Autodesk Fusion 360 part; units mm, degrees
note: some values were not read from the file. Set by a fixed rule: which face or edge a step refers to.
(part 4 of 4)
sketch "Sketch109" plane through (0, 317.5, 0) normal (0, -1, 0) x (1, 0, 0)
  line L0 (-279, 20) -> (-254, 20)
  line L1 (-254, 20) -> (-254, 51.2)
  line L2 (-254, 51.2) -> (-70, 51.2)
  line L3 (-70, 51.2) -> (-70, 76.2)
  line L4 (-70, 76.2) -> (-74.5, 76.2)
  line L5 (-74.5, 76.2) -> (-74.5, 63.7)
  line L6 (-74.5, 63.7) -> (-83.5, 63.7)
  line L7 (-83.5, 63.7) -> (-83.5, 76.2)
  line L8 (-83.5, 76.2) -> (-231.5, 76.2)
  line L9 (-231.5, 76.2) -> (-231.5, 63.7)
  line L10 (-231.5, 63.7) -> (-240.5, 63.7)
  line L11 (-240.5, 63.7) -> (-240.5, 86.2)
  line L12 (-240.5, 86.2) -> (-245, 86.2)
  line L13 (-245, 86.2) -> (-245, 79.7)
  line L14 (-245, 79.7) -> (-314, 79.7)
  line L15 (-314, 79.7) -> (-314, 3)
  line L16 (-314, 3) -> (-279, 3)
  line L17 (-279, 3) -> (-279, 20)
  line L18 (-279, 20) -> (-314, 20)
  line L19 (-314, 20) -> (-314, 3)
  line L20 (-314, 3) -> (-279, 3)
  line L21 (-279, 3) -> (-279, 20)
  constraint horizontal L18
  constraint vertical L19
  constraint horizontal L20
  constraint vertical L21
  constraint coincident L15.end L16.start
  constraint coincident L0.start L17.end
extrude "Extrude276" add sketch "Sketch109" along normal blind 117 separate body contours L15 L16 L17 L18 L19 L20 L21 makes body 17
sketch "Sketch110" plane through (-314, 0, 0) normal (-1, 0, 0) x (0, 0, 1)
  line L0 (20, 317.5) -> (3, 317.5)
  line L1 (3, 317.5) -> (3, 200.5)
  line L2 (3, 200.5) -> (20, 200.5)
  line L3 (20, 200.5) -> (20, 317.5)
  line L4 (20, 200.5) -> (36.1286, 200.5)
  line L5 (36.1286, 200.5) -> (36.1286, 210.5)
  line L6 (36.1286, 210.5) -> (20, 210.5)
  line L7 (20, 210.5) -> (20, 200.5)
  point P0 (36.1286, 210.5)
  constraint horizontal L4
  constraint vertical L5
  constraint horizontal L6
  constraint vertical L7
  constraint coincident P0 L5.end
  constraint coincident L2.end L3.start
extrude "Extrude277" add sketch "Sketch110" against normal blind 35 contours L3 L4 L5 L6 L7 bodies 16 15 17
extrude "Extrude278" cut 1 faces at (-291, 246.1667, 79.7) along direction (0, 0, 1) blind 1 on bodies 16 bodies 16
extrude "Extrude279" cut 1 faces at (-182.1667, 193, 72.0333) along direction (0, 1, 0) blind 7.5 on bodies 16 bodies 16
extrude "Extrude280" add 1 faces at (-294, 210.5, 50.6333) along direction (0, 1, 0) blind 1.5 on bodies 16 bodies 16
extrude "Extrude281" add 1 faces at (-294, 212, 50.6333) along direction (0, 1, 0) blind 2 on bodies 16 bodies 16
extrude "Extrude282" add 1 faces at (-251.6667, 210.5, 15.1667) along direction (0, 1, 0) blind 6.5 on bodies 16 bodies 16
sketch "Sketch111" plane through (-314, 0, 0) normal (-1, 0, 0) x (0, 0, 1)
  line L0 (3, 200.5) -> (86.2, 200.5)
  line L1 (86.2, 200.5) -> (86.2, 333)
  line L2 (86.2, 333) -> (3, 333)
  line L3 (3, 333) -> (3, 200.5)
  line L4 (20, 214) -> (20, 317.5)
  line L5 (20, 317.5) -> (80.7, 317.5)
  line L6 (80.7, 317.5) -> (80.7, 214)
  line L7 (80.7, 214) -> (20, 214)
  line L8 (3, 333) -> (86.2, 333)
  line L9 (86.2, 333) -> (86.2, 200.5)
  line L10 (86.2, 200.5) -> (3, 200.5)
  line L11 (3, 200.5) -> (3, 333)
  constraint horizontal L8
  constraint vertical L9
  constraint horizontal L10
  constraint vertical L11
  constraint coincident L0.end L1.start
  constraint coincident L2.end L3.start
extrude "Extrude283" add sketch "Sketch111" along normal blind 5 separate body contours L0 L1 L2 L3 L8 L9 L10 L11 | L4 L5 L6 L7 makes body 18
extrude "Extrude284" add 1 faces at (-319, 244.6667, 30.7333) along direction (-1, 0, 0) blind 5 on bodies 18 bodies 18
extrude "Extrude285" cut 1 faces at (-294, 249.5, 20) along direction (0, 0, -1) blind 10 on bodies 16 bodies 16
sketch "Sketch112" plane through (0, 0, 0) normal (0, -1, 0) x (1, 0, 0)
  line L0 (-66, -20) -> (-66, -46)
  line L1 (-66, -46) -> (-249, -46)
  line L2 (-249, -46) -> (-249, -20)
  line L3 (-249, -20) -> (-66, -20)
  circle A0 centre (-152, -53.875) radius 4
  circle A1 centre (-163, -12.125) radius 4
  line L4 (-185, 3) -> (-264, 3)
  line L5 (-264, 3) -> (-264, -71)
  line L6 (-264, -71) -> (-56, -71)
  line L7 (-56, -71) -> (-56, 0)
  line L8 (-56, 0) -> (-36, 0)
  line L9 (-36, 0) -> (-36, 36.1286)
  line L10 (-36, 36.1286) -> (-45, 45.1607)
  line L11 (-45, 45.1607) -> (-45, 3)
  line L12 (-45, 3) -> (-130, 3)
  line L13 (-130, 3) -> (-185, 3)
  line L14 (-66, -46) -> (-111, -46)
  line L15 (-111, -46) -> (-111, -20)
  line L16 (-111, -20) -> (-66, -20)
  line L17 (-66, -20) -> (-66, -46)
  line L18 (-249, -46) -> (-204, -46)
  line L19 (-204, -46) -> (-204, -20)
  line L20 (-204, -20) -> (-249, -20)
  line L21 (-249, -20) -> (-249, -46)
  dimension "d708" = 45
  dimension "d709" = 45
  constraint horizontal L14
  constraint vertical L15
  constraint horizontal L16
  constraint vertical L17
  constraint coincident L0.end L1.start
  constraint horizontal L18
  constraint vertical L19
  constraint horizontal L20
  constraint vertical L21
  constraint coincident L1.end L2.start
  measures "d708" distance of L0.end L14.end
  measures "d709" distance of L1.end L18.end
extrude "Extrude286" add sketch "Sketch112" against normal blind 5 separate body contours L0 L1 L3 L14 L15 L16 L17 makes body 19
sketch "Sketch113" plane through (0, 0, 0) normal (0, -1, 0) x (1, 0, 0)
  line L0 (-66, -20) -> (-66, -46)
  line L1 (-66, -46) -> (-249, -46)
  line L2 (-249, -46) -> (-249, -20)
  line L3 (-249, -20) -> (-66, -20)
  circle A0 centre (-152, -53.875) radius 4
  circle A1 centre (-163, -12.125) radius 4
  line L4 (-185, 3) -> (-264, 3)
  line L5 (-264, 3) -> (-264, -71)
  line L6 (-264, -71) -> (-56, -71)
  line L7 (-56, -71) -> (-56, 0)
  line L8 (-56, 0) -> (-36, 0)
  line L9 (-36, 0) -> (-36, 36.1286)
  line L10 (-36, 36.1286) -> (-45, 45.1607)
  line L11 (-45, 45.1607) -> (-45, 3)
  line L12 (-45, 3) -> (-130, 3)
  line L13 (-130, 3) -> (-185, 3)
  line L14 (-249, -20) -> (-204, -20)
  line L15 (-204, -20) -> (-204, -46)
  line L16 (-204, -46) -> (-249, -46)
  line L17 (-249, -46) -> (-249, -20)
  dimension "d712" = 45
  constraint horizontal L14
  constraint vertical L15
  constraint horizontal L16
  constraint vertical L17
  constraint coincident L2.end L3.start
  measures "d712" distance of L2.end L14.end
extrude "Extrude287" add sketch "Sketch113" against normal blind 5 separate body contours L1 L2 L3 L14 L15 L16 L17 makes body 20
sketch "Sketch114" plane through (0, 0, 0) normal (0, 0, -1) x (-1, 0, 0)
  line L0 (36, 333) -> (36, 0)
  line L1 (36, 0) -> (56, 0)
  line L2 (56, 0) -> (56, 328)
  line L3 (56, 328) -> (56, 333)
  line L4 (56, 333) -> (36, 333)
  line L5 (36, 333) -> (56, 333)
  line L6 (56, 333) -> (56, 328)
  line L7 (56, 328) -> (36, 328)
  line L8 (36, 328) -> (36, 333)
  line L9 (56, 328) -> (49.25, 328)
  line L10 (49.25, 328) -> (49.25, 304.4)
  line L11 (49.25, 304.4) -> (56, 304.4)
  line L12 (56, 304.4) -> (56, 328)
  line L13 (49.25, 328) -> (42.75, 328)
  line L14 (42.75, 328) -> (42.75, 304.4)
  line L15 (42.75, 304.4) -> (49.25, 304.4)
  line L16 (49.25, 304.4) -> (49.25, 328)
  dimension "d715" = 6.75
  dimension "d716" = 23.6
  dimension "d717" = 6.5
  constraint horizontal L5
  constraint vertical L6
  constraint horizontal L7
  constraint vertical L8
  constraint coincident L2.end L3.start
  constraint coincident L0.start L4.end
  constraint horizontal L9
  constraint vertical L10
  constraint horizontal L11
  constraint vertical L12
  constraint horizontal L13
  constraint vertical L14
  constraint horizontal L15
  constraint vertical L16
  measures "d715" distance of L2.end L9.end
  measures "d716" distance of L2.end L11.end
  measures "d717" distance of L9.end L13.end
extrude "Extrude288" cut sketch "Sketch114" against normal blind 28 contours L7 L10 L13 L14 L15 L16 bodies 16
sketch "Sketch115" plane through (-56, 0, 0) normal (-1, 0, 0) x (0, 0, 1)
  line L0 (0, 333) -> (0, 328)
  line L1 (0, 328) -> (61.2, 328)
  line L2 (61.2, 328) -> (61.2, 333)
  line L3 (61.2, 333) -> (0, 333)
extrude "Extrude289" cut 1 faces at (-44.9167, 320.1333, 28) along direction (0, 0, 1) blind 5 on bodies 16 bodies 16
sketch "Sketch116" plane through (-61, 0, 0) normal (-1, 0, 0) x (0, 0, 1)
  line L0 (28, 328) -> (33, 328)
  line L1 (33, 328) -> (33, 323)
  line L2 (33, 323) -> (28, 323)
  line L3 (28, 323) -> (28, 328)
  line L4 (28, 323) -> (33, 323)
  line L5 (33, 323) -> (33, 304.4)
  line L6 (33, 304.4) -> (28, 304.4)
  line L7 (28, 304.4) -> (28, 323)
  point P0 (28, 328)
  point P1 (33, 304.4)
  dimension "d725" = 5
  constraint horizontal L0
  constraint vertical L1
  constraint horizontal L2
  constraint vertical L3
  constraint coincident P0 L0.start
  constraint horizontal L4
  constraint vertical L5
  constraint horizontal L6
  constraint vertical L7
  constraint coincident P1 L5.end
  measures "d725" distance of P0 L2.end
extrude "Extrude290" cut sketch "Sketch116" against normal blind 18.25 contours L2 L4 L5 L6 L7 bodies 16
extrude "Extrude291" cut 1 faces at (-245, 70, -59.6667) along direction (0, -1, 0) blind 8 on bodies 16 bodies 16
sketch "Sketch117" plane through (-61, 0, 0) normal (-1, 0, 0) x (0, 0, 1)
  line L0 (0, 304.4) -> (13, 304.4)
  line L1 (13, 304.4) -> (13, 313.4)
  line L2 (13, 313.4) -> (0, 313.4)
  line L3 (0, 313.4) -> (0, 304.4)
  circle A0 centre (13, 313.4) radius 1.375
  point P0 (0, 304.4)
  dimension "d730" = 13
  dimension "d731" = 9
  dimension "d732" = 2.75
  constraint horizontal L0
  constraint vertical L1
  constraint horizontal L2
  constraint vertical L3
  constraint coincident P0 L0.start
  constraint coincident L1.end L2.start
  measures "d730" distance of P0 L0.end
  measures "d731" distance of P0 L2.end
  measures "d732" diameter of A0
extrude "Extrude292" cut sketch "Sketch117" against normal blind 11.75 contours L1 L2 A0 | L1 L2 A0 bodies 16
sketch "Sketch118" plane through (-61, 0, 0) normal (-1, 0, 0) x (0, 0, 1)
  circle A0 centre (13, 313.4) radius 1.375
  circle A1 centre (13, 313.4) radius 1.375
  line L0 (13, 313.4) -> (0, 313.4)
  line L1 (0, 313.4) -> (0, 322.9)
  line L2 (0, 322.9) -> (13, 322.9)
  line L3 (13, 322.9) -> (13, 313.4)
  line L4 (0, 304.4) -> (0, 328)
  circle A2 centre (13, 322.9) radius 1.375
  dimension "d735" = 9.5
  dimension "d736" = 2.75
  constraint concentric A0 A1
  constraint horizontal L0
  constraint vertical L1
  constraint horizontal L2
  constraint vertical L3
  constraint coincident L1.end L4
  constraint coincident A0.centre A1.centre
  constraint coincident L2.end L3.start
  measures "d735" distance of A0.centre L2.end
  measures "d736" diameter of A2
extrude "Extrude293" cut sketch "Sketch118" against normal blind 11.75 contours L2 L3 A2 | L2 L3 A2 bodies 16
sketch "Sketch119" plane through (-61, 0, 0) normal (-1, 0, 0) x (0, 0, 1)
  circle A0 centre (13, 322.9) radius 1.375
  circle A1 centre (13, 322.9) radius 1.375
  circle A2 centre (13, 313.4) radius 1.375
  circle A3 centre (13, 313.4) radius 1.375
  circle A4 centre (13, 322.9) radius 2.375
  circle A5 centre (13, 313.4) radius 2.375
  dimension "d739" = 1
  dimension "d740" = 1
  constraint concentric A0 A1
  constraint concentric A2 A3
extrude "Extrude294" cut sketch "Sketch119" against normal blind 4 bodies 16
extrude "Extrude295" add 1 faces at (-294, 248.5, 10) along direction (0, 0, 1) blind 20 on bodies 16 bodies 16 18
sketch "Sketch120" plane through (0, 200.5, 0) normal (0, -1, 0) x (1, 0, 0)
  line L0 (-279, 3) -> (-279, 36.1286)
  line L1 (-279, 36.1286) -> (-270, 45.1607)
  line L2 (-270, 45.1607) -> (-270, 56.2)
  line L3 (-270, 56.2) -> (-254, 76.2)
  line L4 (-254, 76.2) -> (-254, 56.2)
  line L5 (-254, 56.2) -> (-61, 56.2)
  line L6 (-61, 56.2) -> (-61, 76.2)
  line L7 (-61, 76.2) -> (-74.5, 76.2)
  line L8 (-74.5, 76.2) -> (-74.5, 63.7)
  line L9 (-74.5, 63.7) -> (-83.5, 63.7)
  line L10 (-83.5, 63.7) -> (-83.5, 76.2)
  line L11 (-83.5, 76.2) -> (-231.5, 76.2)
  line L12 (-231.5, 76.2) -> (-231.5, 63.7)
  line L13 (-231.5, 63.7) -> (-240.5, 63.7)
  line L14 (-240.5, 63.7) -> (-240.5, 86.2)
  line L15 (-240.5, 86.2) -> (-324, 86.2)
  line L16 (-324, 86.2) -> (-324, 3)
  line L17 (-324, 3) -> (-279, 3)
  line L18 (-279, 36.1286) -> (-324, 36.1286)
  line L19 (-324, 36.1286) -> (-324, 3)
  line L20 (-324, 3) -> (-279, 3)
  line L21 (-279, 3) -> (-279, 36.1286)
  constraint horizontal L18
  constraint vertical L19
  constraint horizontal L20
  constraint vertical L21
  constraint coincident L16.end L17.start
  constraint coincident L0.end L1.start
extrude "Extrude296" cut sketch "Sketch120" against normal blind 140 contours L0 L16 L17 L18 L19 L20 L21 bodies 16
extrude "Extrude297" add 1 faces at (-305.6667, 327.8333, 36.1286) along direction (0, 0, -1) blind 6.129 on bodies 16 bodies 16
sketch "Sketch121" plane through (0, 0, 29.9996) normal (0, 0, -1) x (-1, 0, 0)
  line L0 (324, 333) -> (279, 333)
  line L1 (279, 333) -> (279, 317.5)
  line L2 (279, 317.5) -> (314, 317.5)
  line L3 (314, 317.5) -> (314, 214)
  line L4 (314, 214) -> (279, 214)
  line L5 (279, 214) -> (279, 200.5)
  line L6 (279, 200.5) -> (324, 200.5)
  line L7 (324, 200.5) -> (324, 333)
  line L8 (279, 333) -> (324, 333)
  line L9 (324, 333) -> (324, 200.5)
  line L10 (324, 200.5) -> (279, 200.5)
  line L11 (279, 200.5) -> (279, 333)
  constraint horizontal L8
  constraint vertical L9
  constraint horizontal L10
  constraint vertical L11
  constraint coincident L6.end L7.start
  constraint coincident L0.end L1.start
extrude "Extrude298" add sketch "Sketch121" along normal blind 5 separate body makes body 21
sketch "Sketch122" plane through (0, 333, 0) normal (0, 1, 0) x (-1, 0, 0)
  line L0 (279, 3) -> (279, 29.9996)
  line L1 (279, 29.9996) -> (324, 29.9996)
  line L2 (324, 29.9996) -> (324, 86.2)
  line L3 (324, 86.2) -> (240.5, 86.2)
  line L4 (240.5, 86.2) -> (240.5, 63.7)
  line L5 (240.5, 63.7) -> (231.5, 63.7)
  line L6 (231.5, 63.7) -> (231.5, 76.2)
  line L7 (231.5, 76.2) -> (83.5, 76.2)
  line L8 (83.5, 76.2) -> (83.5, 63.7)
  line L9 (83.5, 63.7) -> (74.5, 63.7)
  line L10 (74.5, 63.7) -> (74.5, 76.2)
  line L11 (74.5, 76.2) -> (61, 76.2)
  line L12 (61, 76.2) -> (45, 56.1607)
  line L13 (45, 56.1607) -> (53.7273, 56.1821)
  line L14 (53.7273, 56.1821) -> (51, 56.1607)
  line L15 (51, 56.1607) -> (45, 56.1607)
  line L16 (45, 56.1607) -> (45, 45.1607)
  line L17 (45, 45.1607) -> (36, 36.1286)
  line L18 (36, 36.1286) -> (36, 0)
  line L19 (36, 0) -> (56, 0)
  line L20 (56, 0) -> (56, 61.2)
  line L21 (56, 61.2) -> (259, 61.2)
  line L22 (259, 61.2) -> (259, -71)
  line L23 (259, -71) -> (264, -71)
  line L24 (264, -71) -> (264, 3)
  line L25 (264, 3) -> (279, 3)
  line L26 (324, 24.9996) -> (259, 24.9996)
  line L27 (259, 24.9996) -> (259, 86.2)
  line L28 (259, 86.2) -> (324, 86.2)
  line L29 (324, 86.2) -> (324, 24.9996)
  line L30 (324, 86.2) -> (291.5, 86.2)
  line L31 (291.5, 86.2) -> (291.5, 58.1)
  line L32 (291.5, 58.1) -> (324, 58.1)
  line L33 (324, 58.1) -> (324, 86.2)
  line L34 (324, 86.2) -> (307.75, 86.2)
  line L35 (307.75, 86.2) -> (307.75, 72.15)
  line L36 (307.75, 72.15) -> (324, 72.15)
  line L37 (324, 72.15) -> (324, 86.2)
  line L38 (324, 86.2) -> (317, 86.2)
  line L39 (317, 86.2) -> (317, 79.2)
  line L40 (317, 79.2) -> (324, 79.2)
  line L41 (324, 79.2) -> (324, 86.2)
  line L42 (324, 79.2) -> (317, 86.2)
  point P0 (324, 24.9996)
  dimension "d751" = 65
  dimension "d752" = 28.1
  dimension "d753" = 14.05
  dimension "d754" = 7
  dimension "d755" = 7
  constraint horizontal L26
  constraint vertical L27
  constraint horizontal L28
  constraint vertical L29
  constraint coincident L3 L27.end
  constraint coincident P0 L26.start
  constraint horizontal L30
  constraint vertical L31
  constraint horizontal L32
  constraint vertical L33
  constraint coincident L2.end L3.start
  constraint horizontal L34
  constraint vertical L35
  constraint horizontal L36
  constraint vertical L37
  constraint horizontal L38
  constraint vertical L39
  constraint horizontal L40
  constraint vertical L41
  measures "d751" distance of P0 L26.end
  measures "d752" distance of L2.end L32.end
  measures "d753" distance of L2.end L36.end
  measures "d754" distance of L2.end L38.end
  measures "d755" distance of L2.end L40.end
extrude "Extrude299" cut sketch "Sketch122" against normal blind 200 contours L2 L3 L28 L29 L30 L33 L34 L37 L38 L41 L42 bodies 16
sketch "Sketch123" plane through (0, 0, -71) normal (0, 0, -1) x (-1, 0, 0)
  line L0 (259, 333) -> (259, 328)
  line L1 (259, 328) -> (254, 328)
  line L2 (254, 328) -> (254, 25)
  line L3 (254, 25) -> (61, 25)
  line L4 (61, 25) -> (61, 328)
  line L5 (61, 328) -> (56, 328)
  line L6 (56, 328) -> (56, 0)
  line L7 (56, 0) -> (264, 0)
  line L8 (264, 0) -> (264, 333)
  line L9 (264, 333) -> (259, 333)
extrude "Extrude300" add sketch "Sketch123" along normal blind 5 separate body makes body 22
sketch "Sketch124" plane through (-61, 0, 0) normal (-1, 0, 0) x (0, 0, 1)
  circle A0 centre (13, 322.9) radius 2.375
  circle A1 centre (13, 313.4) radius 2.375
  line L0 (33, 323) -> (33, 304.4)
  line L1 (33, 304.4) -> (28, 304.4)
  line L2 (28, 304.4) -> (28, 323)
  line L3 (28, 323) -> (33, 323)
  line L4 (51.2, 5) -> (51.2, 328)
  line L5 (51.2, 328) -> (-71, 328)
  line L6 (-71, 328) -> (-71, 25)
  line L7 (-71, 25) -> (-66, 25)
  line L8 (-66, 25) -> (-66, 217)
  line L9 (-66, 217) -> (-56, 217)
  line L10 (-56, 217) -> (-56, 62)
  line L11 (-56, 62) -> (10, 62)
  line L12 (10, 62) -> (10, 217)
  line L13 (10, 217) -> (20, 217)
  line L14 (20, 217) -> (20, 5)
  line L15 (20, 5) -> (51.2, 5)
extrude "Extrude301" add 1 faces at (-254, 70.1667, 62.8667) along direction (1, 0, 0) blind 10 on bodies 16 bodies 16
extrude "Extrude302" add 1 faces at (-61, 135.3333, 69.5333) along direction (-1, 0, 0) blind 10 on bodies 16 bodies 16
extrude "Extrude303" add 1 faces at (-246.0289, 146, 30.2696) along direction (0, 1, 0) blind 5 on bodies 16 bodies 16
extrude "Extrude304" add 1 faces at (-229.0289, 146, 34.1304) along direction (0, 1, 0) blind 5 on bodies 16 bodies 16
extrude "Extrude305" add 1 faces at (-240.8138, 142, 39.8515) along direction (0, 1, 0) blind 5 on bodies 16 bodies 16
extrude "Extrude306" cut 1 faces at (-235.9784, 135, 39.5909) along direction (0, 1, 0) blind 5 on bodies 16 bodies 16
sketch "Sketch125" plane through (0, 155, 0) normal (0, 1, 0) x (-1, 0, 0)
  line L0 (254, 10) -> (254, 51.2)
  line L1 (254, 51.2) -> (250.5, 51.2)
  line L2 (250.5, 51.2) -> (250.5, 28.7)
  line L3 (250.5, 28.7) -> (226.5, 28.7)
  line L4 (226.5, 28.7) -> (226.5, 51.2)
  line L5 (226.5, 51.2) -> (219, 51.2)
  line L6 (219, 51.2) -> (219, 41.8)
  line L7 (219, 41.8) -> (213.5, 41.8)
  line L8 (213.5, 41.8) -> (213.5, 37.3)
  line L9 (213.5, 37.3) -> (223, 37.3)
  line L10 (223, 37.3) -> (223, 20)
  line L11 (223, 20) -> (236, 20)
  line L12 (236, 20) -> (236, 10)
  line L13 (236, 10) -> (241, 10)
  line L14 (241, 10) -> (241, 15.5)
  line L15 (241, 15.5) -> (247, 15.5)
  line L16 (247, 15.5) -> (247, 10)
  line L17 (247, 10) -> (254, 10)
  line L18 (236, 20) -> (254, 20)
  line L19 (254, 20) -> (254, 10)
  line L20 (254, 10) -> (236, 10)
  line L21 (236, 10) -> (236, 20)
  constraint horizontal L18
  constraint vertical L19
  constraint horizontal L20
  constraint vertical L21
  constraint coincident L0.start L17.end
  constraint coincident L11.end L12.start
extrude "Extrude307" add sketch "Sketch125" along normal blind 62 separate body contours L0 L12 L13 L14 L15 L16 L17 L18 L19 L20 L21 makes body 23
sketch "Sketch126" plane through (0, 333, 0) normal (0, 1, 0) x (-1, 0, 0)
  line L0 (324, 79.2) -> (317, 86.2)
  line L1 (317, 86.2) -> (240.5, 86.2)
  line L2 (240.5, 86.2) -> (240.5, 63.7)
  line L3 (240.5, 63.7) -> (231.5, 63.7)
  line L4 (231.5, 63.7) -> (231.5, 76.2)
  line L5 (231.5, 76.2) -> (83.5, 76.2)
  line L6 (83.5, 76.2) -> (83.5, 63.7)
  line L7 (83.5, 63.7) -> (74.5, 63.7)
  line L8 (74.5, 63.7) -> (74.5, 76.2)
  line L9 (74.5, 76.2) -> (61, 76.2)
  line L10 (61, 76.2) -> (45, 56.1607)
  line L11 (45, 56.1607) -> (53.7273, 56.1821)
  line L12 (53.7273, 56.1821) -> (51, 56.1607)
  line L13 (51, 56.1607) -> (45, 56.1607)
  line L14 (45, 56.1607) -> (45, 45.1607)
  line L15 (45, 45.1607) -> (36, 36.1286)
  line L16 (36, 36.1286) -> (36, 0)
  line L17 (36, 0) -> (56, 0)
  line L18 (56, 0) -> (56, 61.2)
  line L19 (56, 61.2) -> (259, 61.2)
  line L20 (259, 61.2) -> (259, -71)
  line L21 (259, -71) -> (264, -71)
  line L22 (264, -71) -> (264, 3)
  line L23 (264, 3) -> (279, 3)
  line L24 (279, 3) -> (279, 29.9996)
  line L25 (279, 29.9996) -> (324, 29.9996)
  line L26 (324, 29.9996) -> (324, 79.2)
  line L27 (264, 3) -> (259, 3)
  line L28 (259, 3) -> (259, -76)
  line L29 (259, -76) -> (264, -76)
  line L30 (264, -76) -> (264, 3)
  point P0 (259, -76)
  constraint horizontal L27
  constraint vertical L28
  constraint horizontal L29
  constraint vertical L30
  constraint coincident P0 L28.end
  constraint coincident L22.end L23.start
extrude "Extrude308" cut sketch "Sketch126" against normal blind 5 contours L20 L21 L22 L27 L28 L30 bodies 16
extrude "Extrude309" cut 1 faces at (-262.3333, 333, -72.6667) along direction (0, -1, 0) blind 5 on bodies 22 bodies 22
extrude "Extrude310" cut 1 faces at (-264, 179.5, -46.4333) along direction (1, 0, 0) blind 5 on bodies 16 bodies 16
extrude "Extrude311" cut 1 faces at (-264, 109.3333, -72.6667) along direction (1, 0, 0) blind 5 on bodies 22 bodies 22
sketch "Sketch127" plane through (0, 0, 3) normal (0, 0, -1) x (-1, 0, 0)
  line L0 (279, 0) -> (279, 333)
  line L1 (279, 333) -> (259, 333)
  line L2 (259, 333) -> (259, 328)
  line L3 (259, 328) -> (259, 317.5)
  line L4 (259, 317.5) -> (254, 317.5)
  line L5 (254, 317.5) -> (254, 210.5)
  line L6 (254, 210.5) -> (259, 210.5)
  line L7 (259, 210.5) -> (259, 0)
  line L8 (259, 0) -> (185, 0)
  line L9 (185, 0) -> (185, -3)
  line L10 (185, -3) -> (270, -3)
  line L11 (270, -3) -> (270, 0)
  line L12 (270, 0) -> (279, 0)
  line L13 (259, 0) -> (279, 0)
  line L14 (279, 0) -> (279, 333)
  line L15 (279, 333) -> (259, 333)
  line L16 (259, 333) -> (259, 0)
  constraint horizontal L13
  constraint vertical L14
  constraint horizontal L15
  constraint vertical L16
  constraint coincident L0.end L1.start
  constraint coincident L7.end L8.start
extrude "Extrude312" add sketch "Sketch127" along normal blind 3 separate body contours L0 L1 L2 L3 L7 L12 L13 L14 L15 L16 makes body 24
sketch "Sketch128" plane through (0, 333, 0) normal (0, 1, 0) x (-1, 0, 0)
  line L0 (259, 3) -> (279, 3)
  line L1 (279, 3) -> (279, 29.9996)
  line L2 (279, 29.9996) -> (324, 29.9996)
  line L3 (324, 29.9996) -> (324, 79.2)
  line L4 (324, 79.2) -> (317, 86.2)
  line L5 (317, 86.2) -> (240.5, 86.2)
  line L6 (240.5, 86.2) -> (240.5, 63.7)
  line L7 (240.5, 63.7) -> (231.5, 63.7)
  line L8 (231.5, 63.7) -> (231.5, 76.2)
  line L9 (231.5, 76.2) -> (83.5, 76.2)
  line L10 (83.5, 76.2) -> (83.5, 63.7)
  line L11 (83.5, 63.7) -> (74.5, 63.7)
  line L12 (74.5, 63.7) -> (74.5, 76.2)
  line L13 (74.5, 76.2) -> (61, 76.2)
  line L14 (61, 76.2) -> (45, 56.1607)
  line L15 (45, 56.1607) -> (53.7273, 56.1821)
  line L16 (53.7273, 56.1821) -> (51, 56.1607)
  line L17 (51, 56.1607) -> (45, 56.1607)
  line L18 (45, 56.1607) -> (45, 45.1607)
  line L19 (45, 45.1607) -> (36, 36.1286)
  line L20 (36, 36.1286) -> (36, 0)
  line L21 (36, 0) -> (56, 0)
  line L22 (56, 0) -> (56, 61.2)
  line L23 (56, 61.2) -> (259, 61.2)
  line L24 (259, 61.2) -> (259, 3)
  line L25 (56, 61.2) -> (74.5, 61.2)
  line L26 (74.5, 61.2) -> (74.5, 76.2)
  line L27 (74.5, 76.2) -> (56, 76.2)
  line L28 (56, 76.2) -> (56, 61.2)
  line L29 (56, 61.2) -> (56, 76.2)
  line L30 (56, 76.2) -> (51, 76.2)
  line L31 (51, 76.2) -> (51, 61.2)
  line L32 (51, 61.2) -> (56, 61.2)
  line L33 (56, 61.2) -> (56, 76.2)
  line L34 (51, 63.6754) -> (61, 76.2)
  line L35 (51, 61.2) -> (74.5, 61.2)
  line L36 (240.5, 76.2) -> (264, 76.2)
  line L37 (264, 76.2) -> (264, 61.2)
  line L38 (264, 61.2) -> (240.5, 61.2)
  line L39 (240.5, 61.2) -> (240.5, 76.2)
  dimension "d784" = 5
  dimension "d785" = 23.5
  constraint horizontal L25
  constraint vertical L26
  constraint horizontal L27
  constraint vertical L28
  constraint coincident L12.end L13.start
  constraint coincident L22.end L23.start
  constraint vertical L29
  constraint horizontal L30
  constraint vertical L31
  constraint horizontal L32
  constraint vertical L33
  constraint coincident L14 L34.start
  constraint coincident L31 L34.start
  constraint coincident L13.end L14.start
  constraint perpendicular L26 L35
  constraint horizontal L36
  constraint vertical L37
  constraint horizontal L38
  constraint vertical L39
  constraint coincident L6 L36.start
  measures "d784" distance of L27.end L30.end
  measures "d785" distance of L36.start L36.end
extrude "Extrude313" add sketch "Sketch128" along normal blind 5 separate body contours L0 L1 L2 L3 L4 L5 L6 L24 L36 L37 L38 makes body 25
sketch "Sketch129" plane through (0, 333, 0) normal (0, 1, 0) x (-1, 0, 0)
  line L0 (259, 3) -> (279, 3)
  line L1 (279, 3) -> (279, 29.9996)
  line L2 (279, 29.9996) -> (324, 29.9996)
  line L3 (324, 29.9996) -> (324, 79.2)
  line L4 (324, 79.2) -> (317, 86.2)
  line L5 (317, 86.2) -> (240.5, 86.2)
  line L6 (240.5, 86.2) -> (240.5, 63.7)
  line L7 (240.5, 63.7) -> (231.5, 63.7)
  line L8 (231.5, 63.7) -> (231.5, 76.2)
  line L9 (231.5, 76.2) -> (83.5, 76.2)
  line L10 (83.5, 76.2) -> (83.5, 63.7)
  line L11 (83.5, 63.7) -> (74.5, 63.7)
  line L12 (74.5, 63.7) -> (74.5, 76.2)
  line L13 (74.5, 76.2) -> (61, 76.2)
  line L14 (61, 76.2) -> (45, 56.1607)
  line L15 (45, 56.1607) -> (53.7273, 56.1821)
  line L16 (53.7273, 56.1821) -> (51, 56.1607)
  line L17 (51, 56.1607) -> (45, 56.1607)
  line L18 (45, 56.1607) -> (45, 45.1607)
  line L19 (45, 45.1607) -> (36, 36.1286)
  line L20 (36, 36.1286) -> (36, 0)
  line L21 (36, 0) -> (56, 0)
  line L22 (56, 0) -> (56, 61.2)
  line L23 (56, 61.2) -> (259, 61.2)
  line L24 (259, 61.2) -> (259, 3)
  line L25 (49.0235, 61.2) -> (74.5, 61.2)
  line L26 (74.5, 61.2) -> (74.5, 76.2)
  line L27 (74.5, 76.2) -> (49.0235, 76.2)
  line L28 (49.0235, 76.2) -> (49.0235, 61.2)
  line L29 (56, 61.2) -> (51, 61.2)
  line L30 (51, 61.2) -> (51, 76.2)
  line L31 (51, 76.2) -> (56, 76.2)
  line L32 (56, 76.2) -> (56, 61.2)
  line L33 (51, 63.6754) -> (61, 76.2)
  dimension "d788" = 5
  constraint horizontal L25
  constraint vertical L26
  constraint horizontal L27
  constraint vertical L28
  constraint coincident L12.end L13.start
  constraint coincident L14 L25.start
  constraint horizontal L29
  constraint vertical L30
  constraint horizontal L31
  constraint vertical L32
  constraint coincident L22.end L23.start
  constraint coincident L14 L33.start
  constraint coincident L30 L33.start
  constraint coincident L13.end L14.start
  measures "d788" distance of L22.end L29.end
extrude "Extrude314" add sketch "Sketch129" along normal blind 5 separate body contours L14 L18 L19 L20 L21 L22 L25 L29 makes body 26
extrude "Extrude315" add 1 faces at (-265.6667, 334.6667, 3) along direction (0, 0, -1) blind 3 on bodies 25 bodies 25 19 20 21 22 23 26 16 24
extrude "Extrude316" add 1 faces at (-309, 333, 28.3329) along direction (0, 1, 0) blind 5 on bodies 21 bodies 21 26 25
extrude "Extrude317" cut 1 faces at (-56, 334.6667, 20.4) along direction (1, 0, 0) blind 5 on bodies 26 bodies 26
sketch "Sketch130" plane through (0, 333, 0) normal (0, 1, 0) x (-1, 0, 0)
  line L0 (259, 61.2) -> (264, 61.2)
  line L1 (264, 61.2) -> (264, 76.2)
  line L2 (264, 76.2) -> (240.5, 76.2)
  line L3 (240.5, 76.2) -> (240.5, 63.7)
  line L4 (240.5, 63.7) -> (231.5, 63.7)
  line L5 (231.5, 63.7) -> (231.5, 76.2)
  line L6 (231.5, 76.2) -> (83.5, 76.2)
  line L7 (83.5, 76.2) -> (83.5, 63.7)
  line L8 (83.5, 63.7) -> (74.5, 63.7)
  line L9 (74.5, 63.7) -> (74.5, 76.2)
  line L10 (74.5, 76.2) -> (61, 76.2)
  line L11 (61, 76.2) -> (45, 56.1607)
  line L12 (51, 56.1607) -> (45, 56.1607)
  line L13 (45, 56.1607) -> (45, 45.1607)
  line L14 (45, 45.1607) -> (36, 36.1286)
  line L15 (36, 36.1286) -> (36, 0)
  line L16 (36, 0) -> (56, 0)
  line L17 (56, 0) -> (56, 61.2)
  line L18 (56, 61.2) -> (259, 61.2)
  line L19 (56, 0, -5) -> (36, 0, -5)
  line L20 (36, 0, -5) -> (36, 0, 5)
  line L21 (36, 0, 5) -> (56, 0, 5)
  line L22 (56, 0, 5) -> (56, 0, -5)
  line L23 (36, 0, 5) -> (51, 0, 5)
  line L24 (36, 0, -5) -> (43.5, 0, 5)
  line L25 (259, 0, -5) -> (279, 0, -5)
  line L26 (279, 0, -5) -> (279, 0, 5)
  line L27 (279, 0, 5) -> (259, 0, 5)
  line L28 (259, 0, 5) -> (259, 0, -5)
  line L29 (279, 0, -5) -> (269, 0, 5)
  point P0 (56, 0)
  point P1 (36, 0)
  point P2 (259, 0)
  point P3 (279, 0)
  constraint coincident P1 L15.end
  constraint coincident P0 L16.end
extrude "Extrude318" cut sketch "Sketch130" along normal blind 25 contours L16 L20 L24 | L16 L20 L21 L23 L24 | L26 L27 L29 in plane through (0, 333, 0) normal (0, 0, 1) bodies 21 26
extrude "Extrude319" cut 1 faces at (-39.75, 336.3333, 25) along direction (0, 0, 1) blind 21 on bodies 26 bodies 26
extrude "Extrude320" cut 1 faces at (-37.25, 331.3333, 25) along direction (0, 0, 1) blind 19 on bodies 21 bodies 21
sketch "Sketch131" plane through (-259, 0, 0) normal (1, 0, 0) x (0, 0, -1)
  line L0 (0, 338) -> (-61.2, 338)
  line L1 (-61.2, 338) -> (-61.2, 333)
  line L2 (-61.2, 333) -> (-61.2, 328)
  line L3 (-61.2, 328) -> (0, 328)
  line L4 (0, 328) -> (0, 338)
  line L5 (0, 338) -> (-61.2, 338)
  line L6 (-61.2, 338) -> (-61.2, 333)
  line L7 (-61.2, 333) -> (0, 333)
  line L8 (0, 333) -> (0, 338)
  constraint horizontal L5
  constraint vertical L6
  constraint horizontal L7
  constraint vertical L8
  constraint coincident L1.end L2.start
  constraint coincident L0.start L4.end
extrude "Extrude321" cut sketch "Sketch131" against normal blind 5 contours L0 L1 L4 L5 L6 L7 L8 bodies 21
sketch "Sketch132" plane through (0, 338, 0) normal (0, 1, 0) x (-1, 0, 0)
  line L0 (264, 76.2) -> (264, 0)
  line L1 (264, 0) -> (269, 0)
  line L2 (269, 0) -> (269, 25)
  line L3 (269, 25) -> (279, 25)
  line L4 (279, 25) -> (279, 24.9996)
  line L5 (279, 24.9996) -> (324, 24.9996)
  line L6 (324, 24.9996) -> (324, 79.2)
  line L7 (324, 79.2) -> (317, 86.2)
  line L8 (317, 86.2) -> (240.5, 86.2)
  line L9 (240.5, 86.2) -> (240.5, 76.2)
  line L10 (240.5, 76.2) -> (264, 76.2)
  line L11 (324, 24.9996) -> (317, 24.9996)
  line L12 (317, 24.9996) -> (317, 31.9996)
  line L13 (317, 31.9996) -> (324, 31.9996)
  line L14 (324, 31.9996) -> (324, 24.9996)
  line L15 (317, 24.9996) -> (324, 31.9996)
  dimension "d807" = 7
  dimension "d808" = 7
  constraint horizontal L11
  constraint vertical L12
  constraint horizontal L13
  constraint vertical L14
  constraint coincident L5.end L6.start
  measures "d807" distance of L5.end L11.end
  measures "d808" distance of L5.end L13.end
extrude "Extrude322" cut sketch "Sketch132" against normal blind 140 contours L5 L6 L11 L14 L15 bodies 21
sketch "Sketch133" plane through (0, 0, 0) normal (0, 0, -1) x (-1, 0, 0)
  line L0 (43.5, 338) -> (39.75, 333)
  line L1 (39.75, 333) -> (51, 333)
  line L2 (51, 333) -> (51, 338)
  line L3 (51, 338) -> (43.5, 338)
  line L4 (39.75, 333) -> (42.65, 333)
  line L5 (42.65, 333) -> (42.65, 338)
  line L6 (42.65, 338) -> (39.75, 338)
  line L7 (39.75, 338) -> (39.75, 333)
  line L8 (42.65, 333) -> (51, 333)
  line L9 (51, 333) -> (51, 338)
  line L10 (51, 338) -> (42.65, 338)
  line L11 (42.65, 338) -> (42.65, 333)
  line L12 (51, 333) -> (46, 333)
  line L13 (46, 333) -> (46, 338)
  line L14 (46, 338) -> (51, 338)
  line L15 (51, 338) -> (51, 333)
  line L16 (46, 338) -> (51, 338)
  line L17 (51, 338, 0) -> (51, 338, -61.2)
  line L18 (51, 338, -61.2) -> (46, 338, -61.2)
  line L19 (46, 338, -61.2) -> (46, 338, 0)
  line L20 (46, 338) -> (51, 338)
  line L21 (51, 338) -> (51, 343)
  line L22 (51, 343) -> (46, 343)
  line L23 (46, 343) -> (46, 338)
  line L24 (51, 343) -> (46, 338)
  point P0 (51, 338)
  dimension "d811" = 2.9
  dimension "d812" = 5
  dimension "d813" = 5
  constraint horizontal L4
  constraint vertical L5
  constraint horizontal L6
  constraint vertical L7
  constraint coincident L0.end L1.start
  constraint horizontal L8
  constraint vertical L9
  constraint horizontal L10
  constraint vertical L11
  constraint coincident P0 L2.end
  constraint horizontal L12
  constraint vertical L13
  constraint horizontal L14
  constraint vertical L15
  constraint coincident L1.end L2.start
  constraint horizontal L16
  constraint horizontal L20
  constraint vertical L21
  constraint horizontal L22
  constraint vertical L23
  measures "d811" distance of L0.end L4.end
  measures "d812" distance of L1.end L12.end
  measures "d813" distance of L13.end L22.end
extrude "Extrude323" add sketch "Sketch133" against normal blind 61.2 separate body contours L3 L10 L14 L16 L20 L21 L24 makes body 27
sketch "Sketch134" plane through (0, 338, 0) normal (0, -1, 0) x (1, 0, 0)
  line L0 (-51, 0) -> (-46, 0)
  line L1 (-46, 0) -> (-46, 61.2)
  line L2 (-46, 61.2) -> (-51, 61.2)
  line L3 (-51, 61.2) -> (-51, 0)
  line L4 (-49.0235, 61.2) -> (-46, 57.4132)
  line L5 (-46, 61.2) -> (-46, 57.4132)
  line L6 (-49.0235, 61.2) -> (-46, 61.2)
  point P0 (-49.0235, 61.2)
  constraint coincident P0 L4.start
  constraint coincident L1 L4.end
  constraint coincident L1.end L2.start
  constraint perpendicular L2 L5
extrude "Extrude324" cut sketch "Sketch134" against normal blind 7 contours L1 L2 L4 L5 L6 bodies 27
sketch "Sketch135" plane through (0, 0, 0) normal (0, 0, -1) x (-1, 0, 0)
  line L0 (264, 338) -> (264, 333)
  line L1 (264, 333) -> (259, 333)
  line L2 (259, 333) -> (259, 328)
  line L3 (259, 328) -> (259, 0)
  line L4 (259, 0) -> (279, 0)
  line L5 (279, 0) -> (279, 328)
  line L6 (279, 328) -> (269, 338)
  line L7 (269, 338) -> (264, 338)
  line L8 (264, 338) -> (259, 338)
  line L9 (259, 338) -> (259, 343)
  line L10 (259, 343) -> (264, 343)
  line L11 (264, 343) -> (264, 338)
  line L12 (269, 338) -> (279, 338)
  line L13 (279, 338) -> (279, 328)
  line L14 (279, 328) -> (269, 328)
  line L15 (269, 328) -> (269, 338)
  line L16 (269, 328) -> (274, 328)
  line L17 (274, 328) -> (274, 333)
  line L18 (274, 333) -> (269, 333)
  line L19 (269, 333) -> (269, 328)
  dimension "d818" = 5
  dimension "d819" = 5
  constraint horizontal L8
  constraint vertical L9
  constraint horizontal L10
  constraint vertical L11
  constraint coincident L0.start L7.end
  constraint horizontal L12
  constraint vertical L13
  constraint horizontal L14
  constraint vertical L15
  constraint coincident L5.end L6.start
  constraint coincident L6.end L7.start
  constraint horizontal L16
  constraint vertical L17
  constraint horizontal L18
  constraint vertical L19
  constraint midpoint L6 L17.end
  measures "d818" distance of L0.start L8.end
  measures "d819" distance of L0.start L10.end
extrude "Extrude325" cut sketch "Sketch135" against normal blind 25 contours L6 L15 L18 bodies 21
sketch "Sketch136" plane through (0, 0, 0) normal (0, 0, -1) x (-1, 0, 0)
  line L0 (274, 333) -> (269, 333)
  line L1 (269, 333) -> (269, 338)
  line L2 (269, 338) -> (264, 338)
  line L3 (264, 338) -> (264, 333)
  line L4 (264, 333) -> (259, 333)
  line L5 (259, 333) -> (259, 328)
  line L6 (259, 328) -> (259, 0)
  line L7 (259, 0) -> (279, 0)
  line L8 (279, 0) -> (279, 328)
  line L9 (279, 328) -> (274, 333)
  line L10 (264, 338) -> (269, 338)
  line L11 (269, 338) -> (269, 343)
  line L12 (269, 343) -> (264, 343)
  line L13 (264, 343) -> (264, 338)
  line L14 (264, 343) -> (269, 338)
  dimension "d822" = 5
  dimension "d823" = 5
  constraint horizontal L10
  constraint vertical L11
  constraint horizontal L12
  constraint vertical L13
  constraint coincident L2.end L3.start
  measures "d822" distance of L2.end L1.end
  measures "d823" distance of L2.end L12.end
extrude "Extrude326" add sketch "Sketch136" against normal blind 86.2 separate body contours L2 L10 L13 L14 makes body 28
sketch "Sketch137" plane through (0, 333, 0) normal (0, 1, 0) x (-1, 0, 0)
  line L0 (39.75, 39.892) -> (39.75, 0)
  line L1 (39.75, 0) -> (56, 0)
  line L2 (56, 0) -> (56, 61.2)
  line L3 (56, 61.2) -> (259, 61.2)
  line L4 (259, 61.2) -> (259, 0)
  line L5 (259, 0) -> (264, 0)
  line L6 (264, 0) -> (264, 76.2)
  line L7 (264, 76.2) -> (240.5, 76.2)
  line L8 (240.5, 76.2) -> (240.5, 63.7)
  line L9 (240.5, 63.7) -> (231.5, 63.7)
  line L10 (231.5, 63.7) -> (231.5, 76.2)
  line L11 (231.5, 76.2) -> (83.5, 76.2)
  line L12 (83.5, 76.2) -> (83.5, 63.7)
  line L13 (83.5, 63.7) -> (74.5, 63.7)
  line L14 (74.5, 63.7) -> (74.5, 76.2)
  line L15 (74.5, 76.2) -> (61, 76.2)
  line L16 (61, 76.2) -> (45, 56.1607)
  line L17 (45, 56.1607) -> (53.7273, 56.1821)
  line L18 (53.7273, 56.1821) -> (51, 56.1607)
  line L19 (51, 56.1607) -> (45, 56.1607)
  line L20 (45, 56.1607) -> (45, 45.1607)
  line L21 (45, 45.1607) -> (39.75, 39.892)
  line L22 (264, 61.2) -> (264, 86.2)
  line L23 (264, 86.2, 0) -> (264, 86.2, 10)
  line L24 (264, 86.2, 10) -> (264, 61.2, 10)
  line L25 (264, 61.2, 10) -> (264, 61.2, 0)
  line L26 (269, 86.2, 5) -> (264, 86.2, 10)
  line L27 (269, 86.2, 5) -> (264, 86.2, 5)
  point P0 (264, 86.2)
  point P1 (269, 86.2)
  point P2 (264, 86.2)
  constraint vertical L22
  constraint coincident P2 P0
  constraint coincident L6 L22.start
extrude "Extrude327" cut sketch "Sketch137" against normal blind 25 contours L23 L26 L27 in plane through (0, 333, 86.2) normal (0, 0, 1) bodies 28
sketch "Sketch138" plane through (-264, 0, 0) normal (1, 0, 0) x (0, 0, -1)
  line L0 (-61.2, 343) -> (-61.2, 338)
  line L1 (-61.2, 338) -> (0, 338)
  line L2 (0, 338) -> (0, 343)
  line L3 (0, 343) -> (-61.2, 343)
  line L4 (-61.2, 338) -> (-56.2, 338)
  line L5 (-56.2, 338) -> (-56.2, 343)
  line L6 (-56.2, 343) -> (-61.2, 343)
  line L7 (-61.2, 343) -> (-61.2, 338)
  line L8 (-56.2, 343) -> (-61.2, 343)
  line L9 (-61.2, 343, 0) -> (-61.2, 343, -5)
  line L10 (-61.2, 343, -5) -> (-56.2, 343, -5)
  line L11 (-56.2, 343, -5) -> (-56.2, 343, 0)
  line L12 (-56.2, 343, -5) -> (-61.2, 343, 0)
  dimension "d828" = 5
  dimension "d829" = 5
  dimension "d830" = 5
  dimension "d831" = 5
  constraint horizontal L4
  constraint vertical L5
  constraint horizontal L6
  constraint vertical L7
  constraint coincident L0.end L1.start
  constraint horizontal L8
  measures "d828" distance of L0.end L4.end
  measures "d829" distance of L0.end L0.start
  measures "d830" distance of L5.end L0.start
  measures "d831" distance of L5.end L6.start
extrude "Extrude328" cut sketch "Sketch138" against normal blind 5 contours L9 L10 L12 in plane through (-264, 343, 0) normal (0, 1, 0) bodies 28
sketch "Sketch139" plane through (-240.5, 0, 0) normal (1, 0, 0) x (0, 0, -1)
  line L0 (-76.2, 333) -> (-76.2, 338)
  line L1 (-76.2, 338) -> (-86.2, 338)
  line L2 (-86.2, 338) -> (-86.2, 317.5)
  line L3 (-86.2, 317.5) -> (-63.7, 317.5)
  line L4 (-63.7, 317.5) -> (-63.7, 333)
  line L5 (-63.7, 333) -> (-76.2, 333)
  line L6 (-86.2, 338) -> (-81.2, 338)
  line L7 (-81.2, 338) -> (-81.2, 333)
  line L8 (-81.2, 333) -> (-86.2, 333)
  line L9 (-86.2, 333) -> (-86.2, 338)
  line L10 (-81.2, 338) -> (-86.2, 333)
  dimension "d834" = 5
  dimension "d835" = 5
  constraint horizontal L6
  constraint vertical L7
  constraint horizontal L8
  constraint vertical L9
  constraint coincident L1.end L2.start
  measures "d834" distance of L1.end L6.end
  measures "d835" distance of L1.end L8.end
extrude "Extrude329" cut sketch "Sketch139" against normal blind 112 contours L1 L2 L6 L9 L10 bodies 21
sketch "Sketch140" plane through (-240.5, 0, 0) normal (1, 0, 0) x (0, 0, -1)
  line L0 (-86.2, 200.5) -> (-63.7, 200.5)
  line L1 (-63.7, 200.5) -> (-63.7, 214)
  line L2 (-63.7, 214) -> (-86.2, 214)
  line L3 (-86.2, 214) -> (-86.2, 200.5)
  line L4 (-86.2, 200.5) -> (-81.2, 200.5)
  line L5 (-81.2, 200.5) -> (-81.2, 205.5)
  line L6 (-81.2, 205.5) -> (-86.2, 205.5)
  line L7 (-86.2, 205.5) -> (-86.2, 200.5)
  line L8 (-86.2, 205.5) -> (-81.2, 200.5)
  dimension "d838" = 5
  dimension "d839" = 5
  constraint horizontal L4
  constraint vertical L5
  constraint horizontal L6
  constraint vertical L7
  constraint coincident L0.start L3.end
  measures "d838" distance of L0.start L4.end
  measures "d839" distance of L0.start L6.end
extrude "Extrude330" cut sketch "Sketch140" against normal blind 97 contours L0 L3 L4 L7 L8 bodies 21
sketch "Sketch141" plane through (0, 0, 86.2) normal (0, 0, 1) x (1, 0, 0)
  line L0 (-317, 205.5) -> (-240.5, 205.5)
  line L1 (-240.5, 205.5) -> (-240.5, 214)
  line L2 (-240.5, 214) -> (-245, 214)
  line L3 (-245, 214) -> (-245, 317.5)
  line L4 (-245, 317.5) -> (-240.5, 317.5)
  line L5 (-240.5, 317.5) -> (-240.5, 333)
  line L6 (-240.5, 333) -> (-317, 333)
  line L7 (-317, 333) -> (-317, 205.5)
  line L8 (-317, 205.5) -> (-322, 205.5)
  line L9 (-322, 205.5) -> (-322, 200.5)
  line L10 (-322, 200.5) -> (-317, 200.5)
  line L11 (-317, 200.5) -> (-317, 205.5)
  line L12 (-317, 200.5) -> (-322, 205.5)
  dimension "d842" = 5
  dimension "d843" = 5
  constraint horizontal L8
  constraint vertical L9
  constraint horizontal L10
  constraint vertical L11
  constraint coincident L0.start L7.end
  measures "d842" distance of L0.start L8.end
  measures "d843" distance of L0.start L10.end
extrude "Extrude331" cut sketch "Sketch141" against normal blind 70 contours L9 L10 L12 bodies 21
extrude "Extrude332" cut 1 faces at (-322, 202.1667, 64.1332) along direction (-1, 0, 0) blind 3 on bodies 21 bodies 21
extrude "Extrude333" cut 1 faces at (-322.6667, 205.5, 47.733) along direction (0, 1, 0) blind 195 on bodies 21 bodies 21
sketch "Sketch142" plane through (0, 0, 24.9996) normal (0, 0, -1) x (-1, 0, 0)
  line L0 (317, 200.5) -> (317, 338)
  line L1 (317, 338) -> (279, 338)
  line L2 (279, 338) -> (279, 328)
  line L3 (279, 328) -> (279, 200.5)
  line L4 (279, 200.5) -> (317, 200.5)
  line L5 (317, 338) -> (322, 338)
  line L6 (322, 338) -> (322, 333)
  line L7 (322, 333) -> (317, 333)
  line L8 (317, 333) -> (317, 338)
  line L9 (317, 338) -> (322, 333)
  dimension "d850" = 5
  dimension "d851" = 5
  constraint horizontal L5
  constraint vertical L6
  constraint horizontal L7
  constraint vertical L8
  constraint coincident L0.end L1.start
  measures "d850" distance of L0.end L5.end
  measures "d851" distance of L0.end L7.end
extrude "Extrude334" cut sketch "Sketch142" against normal blind 70 contours L5 L6 L9 bodies 21
sketch "Sketch143" plane through (-322, 0, 0) normal (-1, 0, 0) x (0, 0, 1)
  line L0 (81.2, 333) -> (29.9996, 333)
  line L1 (29.9996, 333) -> (29.9996, 205.5)
  line L2 (29.9996, 205.5) -> (81.2, 205.5)
  line L3 (81.2, 205.5) -> (81.2, 333)
  line L4 (29.9996, 333) -> (24.9996, 333)
  line L5 (24.9996, 333) -> (24.9996, 338)
  line L6 (24.9996, 338) -> (29.9996, 338)
  line L7 (29.9996, 338) -> (29.9996, 333)
  line L8 (24.9996, 333) -> (29.9996, 338)
  dimension "d854" = 5
  dimension "d855" = 5
  constraint horizontal L4
  constraint vertical L5
  constraint horizontal L6
  constraint vertical L7
  constraint coincident L0.end L1.start
  measures "d854" distance of L0.end L4.end
  measures "d855" distance of L0.end L6.end
extrude "Extrude335" cut sketch "Sketch143" against normal blind 53 contours L5 L6 L8 bodies 21
sketch "Sketch144" plane through (-322, 0, 0) normal (-1, 0, 0) x (0, 0, 1)
  line L0 (81.2, 333) -> (29.9996, 333)
  line L1 (29.9996, 333) -> (29.9996, 205.5)
  line L2 (29.9996, 205.5) -> (81.2, 205.5)
  line L3 (81.2, 205.5) -> (81.2, 333)
  line L4 (29.9996, 205.5) -> (24.9996, 205.5)
  line L5 (24.9996, 205.5) -> (24.9996, 200.5)
  line L6 (24.9996, 200.5) -> (29.9996, 200.5)
  line L7 (29.9996, 200.5) -> (29.9996, 205.5)
  line L8 (24.9996, 205.5) -> (29.9996, 200.5)
  dimension "d858" = 5
  dimension "d859" = 5
  constraint horizontal L4
  constraint vertical L5
  constraint horizontal L6
  constraint vertical L7
  constraint coincident L1.end L2.start
  measures "d858" distance of L1.end L4.end
  measures "d859" distance of L1.end L6.end
extrude "Extrude336" cut sketch "Sketch144" against normal blind 43 contours L5 L6 L8 bodies 21
sketch "Sketch145" plane through (0, 0, 86.2) normal (0, 0, 1) x (1, 0, 0)
  line L0 (-317, 205.5) -> (-240.5, 205.5)
  line L1 (-240.5, 205.5) -> (-240.5, 214)
  line L2 (-240.5, 214) -> (-245, 214)
  line L3 (-245, 214) -> (-245, 317.5)
  line L4 (-245, 317.5) -> (-240.5, 317.5)
  line L5 (-240.5, 317.5) -> (-240.5, 333)
  line L6 (-240.5, 333) -> (-317, 333)
  line L7 (-317, 333) -> (-317, 205.5)
  line L8 (-264, 338, -25) -> (-269, 338, -25)
  line L9 (-264, 343, -25) -> (-264, 338, -25)
  line L10 (-269, 338, -30) -> (-269, 338, -25)
  line L11 (-269, 338, -30) -> (-264, 343, -25)
  line L12 (-269, 338, -25) -> (-264, 343, -25)
  point P0 (-264, 338)
  point P1 (-269, 338)
  dimension "d862" = 5
  dimension "d863" = 5
  measures "d862" distance of P0 P1
extrude "Extrude337" add sketch "Sketch145" along normal blind 15 separate body contours L8 L9 L12 in plane through (0, 0, 61.2) normal (0, 0, 1) makes body 29
sketch "Sketch146" plane through (0, 338, 0) normal (0, 1, 0) x (-1, 0, 0)
  line L0 (269, 29.9996) -> (317, 29.9996)
  line L1 (317, 29.9996) -> (317, 81.2)
  line L2 (317, 81.2) -> (240.5, 81.2)
  line L3 (240.5, 81.2) -> (240.5, 76.2)
  line L4 (240.5, 76.2) -> (264, 76.2)
  line L5 (264, 76.2) -> (264, 0)
  line L6 (264, 0) -> (269, 0)
  line L7 (269, 0) -> (269, 29.9996)
  line L8 (269, 61.2) -> (269, 56.2)
  line L9 (269, 56.2) -> (264, 61.2)
  line L10 (269, 61.2) -> (264, 61.2)
  point P0 (269, 61.2)
  point P1 (269, 56.2)
  point P2 (264, 61.2)
  constraint coincident P0 L8.start
  constraint coincident P1 L8.end
  constraint coincident P2 L9.end
extrude "Extrude338" add sketch "Sketch146" along normal blind 5 contours L8 L9 L10 bodies 28 22 23 26 27 21 29
extrude "Extrude339" cut 1 faces at (-267.3333, 341.3333, 61.2) along direction (0, 0, -1) blind 8 on bodies 28 bodies 28
sketch "Sketch147" plane through (0, 338, 0) normal (0, 1, 0) x (-1, 0, 0)
  line L0 (269, 76.2) -> (269, 29.9996)
  line L1 (269, 29.9996) -> (317, 29.9996)
  line L2 (317, 29.9996) -> (317, 81.2)
  line L3 (317, 81.2) -> (240.5, 81.2)
  line L4 (240.5, 81.2) -> (240.5, 76.2)
  line L5 (240.5, 76.2) -> (264, 76.2)
  line L6 (264, 76.2) -> (269, 76.2)
  line L7 (264, 76.2, 5) -> (269, 76.2, 5)
  line L8 (269, 76.2, 5) -> (269, 71.2, 5)
  line L9 (269, 71.2, 5) -> (264, 71.2, 5)
  line L10 (264, 71.2, 5) -> (264, 76.2, 5)
  line L11 (264, 76.2, 5) -> (269, 71.2, 5)
  point P0 (264, 76.2)
  dimension "d870" = 5
  dimension "d871" = 5
  constraint coincident P0 L5.end
  measures "d870" distance of P0 L0.start
extrude "Extrude340" cut sketch "Sketch147" against normal blind 5 contours L7 L8 L11 in plane through (0, 343, 0) normal (0, 1, 0) bodies 28
extrude "Extrude341" cut 1 faces at (-68, 165.3333, 13.6667) along direction (1, 0, 0) blind 3.5 on bodies 28 bodies 28
extrude "Extrude342" cut 1 faces at (-68, 113.6667, -59.6667) along direction (1, 0, 0) blind 3.5 on bodies 28 bodies 28
extrude "Extrude343" add 1 faces at (-74, 165.3333, -59.6667) along direction (1, 0, 0) blind 3.5 on bodies 28 bodies 28
extrude "Extrude344" add 1 faces at (-74, 165.3333, 13.6667) along direction (1, 0, 0) blind 3.5 on bodies 28 bodies 28
